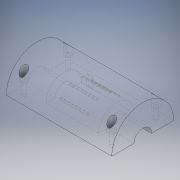
# Autodesk Inventor part: Slider Mount_C
Saved by Autodesk Inventor 2018 (Build 220112000, 112)
## iProperties
Created: 2018-01-08
Part Number: Slider Mount_C
Material: Generic
Document SubType Name: Modeling
Designer: njcfu
Density: 1 g/cm^3
Appearance: Default
Author: njcfu
Autodesk Inventor part; units mm, degrees
ref_plane "YZ Plane" through (0, 0, 0) normal (1, 0, 0) x (0, 1, 0)
ref_plane "XY Plane" through (0, 0, 0) normal (0, 0, 1) x (1, 0, 0)
sketch "Sketch1" plane through (0, 0, 0) normal (1, 0, 0) x (0, 1, 0)
  arc A0 (0, -25.4) -> (0, 25.4) centre (0, 0) ccw
  arc A1 (0, -44.45) -> (0, 44.45) centre (0, 0) ccw
  line L0 (0, 44.45) -> (0, 25.4)
  line L1 (0, -25.4) -> (0, -44.45)
  dimension "d24" = 25.4
  dimension "d27" = 44.45
  dimension "d29" = 0
  dimension "d32" = 19.05
  constraints: 4 end point, 4 point on circle, 2 centre point, 2 coincident, 1 collinear, 1 vertical
  measures "d24" distance of A0.centre L0.end
  measures "d27" radius of A1
  measures "d29" distance from line of point (0, 0) L1
  measures "d32" distance of L0.start L0.end
extrude "Extrusion1" add sketch "Sketch1" along normal mid plane 49.9999
ref_plane "Work Plane2" through (0, 25.4, 0) normal (0, 1, 0) x (-1, 0, 0)
sketch "Sketch3" plane through (0, 25.4, 0) normal (0, 1, 0) x (-1, 0, 0)
  point P0 (0, 0)
sketch "Sketch4" plane through (0, 25.4, 0) normal (0, 1, 0) x (-1, 0, 0)
  line L0 (3.3655, 0.9525) -> (-3.3655, 0.9525)
  line L1 (-3.3655, 0.9525) -> (-3.3655, -0.9525)
  line L2 (-3.3655, -0.9525) -> (3.3655, -0.9525)
  line L3 (3.3655, -0.9525) -> (3.3655, 0.9525)
  line L4 (3.3655, 0.9525) -> (-3.3655, -0.9525) construction
  line L5 (-3.3655, 0.9525) -> (3.3655, -0.9525) construction
  point P0 (0, 0)
  dimension "d30" = 6.731
  dimension "d31" = 1.905
  constraints: 12 end point, 2 midpoint, 2 parallel, 1 horizontal, 1 perpendicular
  measures "d30" distance of L1.end L2.end
  measures "d31" distance of L2.end L0.start
extrude "Extrusion3" cut sketch "Sketch4" along normal blind 14.986 and the other way blind 1.27
sketch "Sketch5" plane through (-25, 0, 0) normal (-1, 0, 0) x (0, 0, 1)
  arc A0 (44.45, 0) -> (-44.45, 0) centre (0, 0) ccw
  arc A1 (25.4, 0) -> (-25.4, 0) centre (0, 0) ccw
  arc A2 (44.45, 0) -> (-44.45, 0) centre (0, 0) ccw projected
  line L0 (-44.45, 0) -> (-25.4, 0) projected
  line L1 (-44.45, 0) -> (-25.4, 0)
  line L2 (25.4, 0) -> (44.45, 0)
  dimension "d40" = 19.05
  constraints: 4 end point, 4 point on circle, 2 centre point, 2 coincident, 2 collinear
  measures "d40" distance of L2.start L2.end
extrude "Extrusion4" add sketch "Sketch5" along normal blind 12.7
sketch "Sketch6" plane through (25, 0, 0) normal (1, 0, 0) x (0, 0, -1)
  arc A0 (44.45, 0) -> (-44.45, 0) centre (0, 0) ccw
  arc A1 (25.4, 0) -> (-25.4, 0) centre (0, 0) ccw
  line L0 (-44.45, 0) -> (-25.4, 0)
  line L1 (25.4, 0) -> (44.45, 0)
  dimension "d43" = 44.45
  dimension "d44" = 25.4
  dimension "d45" = 19.05
  dimension "d46" = 19.05
  constraints: 4 end point, 4 point on circle, 2 centre point, 2 coincident, 2 horizontal
  measures "d43" radius of A0
  measures "d44" radius of A1
  measures "d45" distance of L0.start L0.end
  measures "d46" distance of L1.start L1.end
extrude "Extrusion5" add sketch "Sketch6" along normal blind 12.7
sketch "Sketch7" plane through (-37.7, 0, 0) normal (-1, 0, 0) x (0, 0, 1)
  arc A0 (44.45, 0) -> (-44.45, 0) centre (0, 0) ccw
  arc A1 (12.7, 0) -> (-12.7, 0) centre (0, 0) ccw
  line L0 (-44.45, 0) -> (-12.7, 0)
  line L1 (12.7, 0) -> (44.45, 0)
  dimension "d49" = 44.45
  dimension "d50" = 12.7
  dimension "d51" = 31.75
  constraints: 4 end point, 4 point on circle, 2 centre point, 2 coincident, 2 point on line, 1 horizontal
  measures "d49" radius of A0
  measures "d50" radius of A1
  measures "d51" distance of L0.start L0.end
extrude "Extrusion6" add sketch "Sketch7" along normal blind 38.1
sketch "Sketch8" plane through (0, 0, 0) normal (1, 0, 0) x (0, 1, 0)
  line L0 (0, 0) -> (12.7, 21.997)
  line L1 (12.7, 21.997) -> (13.7999, 21.362)
  line L2 (13.7999, 21.362) -> (14.4349, 22.4619)
  line L3 (14.4349, 22.4619) -> (12.2351, 23.7319)
  line L4 (12.2351, 23.7319) -> (11.6001, 22.632)
  line L5 (11.6001, 22.632) -> (12.7, 21.997)
  line L6 (11.6001, 22.632) -> (11.2826, 22.0821)
  line L7 (11.2826, 22.0821) -> (13.4824, 20.8121)
  line L8 (13.4824, 20.8121) -> (13.7999, 21.362)
  line L9 (0, -12.7) -> (0, -25.4) projected
  dimension "d55" = 2.54
  dimension "d56" = 1.27
  dimension "d57" = 0.635
  dimension "d58" = 1.27
  dimension "d59" = 210
  dimension "d60" = 25.4
  constraints: 18 end point, 7 perpendicular, 1 collinear
  measures "d55" distance of L6.end L7.end
  measures "d56" distance between parallel lines of L0 L6
  measures "d57" distance between parallel lines of L7 L5
  measures "d58" distance between parallel lines of L5 L3
  measures "d60" distance of L0.start L0.end
extrude "Extrusion7" cut sketch "Sketch8" along normal mid plane 39.9999
pattern_circular "Circular Pattern2" count 4 over 120 about axis through (-10, 0, 0) along (-1, 0, 0) of "Extrusion7"
fillet "Fillet5" radius 0.254 8 edges at (0, 12.2351, -23.7319) (0, 14.4349, -22.4619) (0, 24.6272, -10.3151) (0, 25.496, -7.9283) (0, 25.496, 7.9283) (0, 24.6272, 10.3151) (0, 14.4349, 22.4619) (0, 12.2351, 23.7319)
sketch "Sketch9" plane through (37.7, 0, 0) normal (1, 0, 0) x (0, 0, -1)
  arc A0 (44.45, 0) -> (-44.45, 0) centre (0, 0) ccw
  arc A1 (12.7, 0) -> (-12.7, 0) centre (0, 0) ccw
  line L0 (-44.45, 0) -> (-12.7, 0)
  line L1 (12.7, 0) -> (44.45, 0)
  dimension "d67" = 44.45
  dimension "d68" = 12.7
  dimension "d69" = 31.75
  dimension "d70" = 12.7
  dimension "d71" = 44.45
  constraints: 4 end point, 4 point on circle, 2 centre point, 2 coincident, 2 point on line, 1 horizontal
  measures "d67" radius of A0
  measures "d68" radius of A1
  measures "d69" distance of L0.start L0.end
  measures "d70" distance of L0.end point (0, 0)
  measures "d71" distance of L1.end point (0, 0)
extrude "Extrusion8" add sketch "Sketch9" along normal blind 38.1
sketch "Sketch10" plane through (-37.7, 0, 12.7) normal (0, -1, 0) x (1, 0, 0)
  circle A0 centre (100.7999, 19.05) radius 2.413
  circle A1 centre (100.7999, -44.45) radius 2.413
  circle A2 centre (-25.4, -44.45) radius 2.413
  circle A3 centre (-25.4, 19.05) radius 2.413
  line L0 (113.4999, 31.75) -> (113.4999, 0) projected
  line L1 (-38.1, 31.75) -> (113.4999, 31.75) projected
  line L2 (-38.1, -57.15) -> (113.4999, -57.15) projected
  line L3 (113.4999, -25.4) -> (113.4999, -57.15) projected
  line L4 (-38.1, 0) -> (-38.1, 31.75) projected
  line L5 (-38.1, -57.15) -> (-38.1, -25.4) projected
  point P0 (37.6999, -12.7)
  dimension "d74" = 4.826
  dimension "d75" = 12.7
  dimension "d76" = 12.7
  dimension "d77" = 12.7
  dimension "d78" = 12.7
  dimension "d79" = 4.826
  dimension "d80" = 12.7
  dimension "d81" = 12.7
  dimension "d82" = 12.7
  dimension "d83" = 12.7
  dimension "d84" = 4.826
  dimension "d85" = 4.826
  constraints: 4 centre point
  measures "d74" diameter of A0
  measures "d75" distance from line of L0 A0.centre
  measures "d76" distance from line of L1 A0.centre
  measures "d77" distance from line of L2 A1.centre
  measures "d78" distance from line of L3 A1.centre
  measures "d79" diameter of A1
  measures "d80" distance from line of L1 A3.centre
  measures "d81" distance from line of L4 A3.centre
  measures "d82" distance from line of L5 A2.centre
  measures "d83" distance from line of L2 A2.centre
  measures "d84" diameter of A2
  measures "d85" diameter of A3
extrude "Extrusion9" cut sketch "Sketch10" against normal blind 38.1
ref_plane "Work Plane3" through (-37.7, 28.4375, 12.7) normal (0, -1, 0) x (1, 0, 0)
sketch "Sketch11" plane through (-37.7, 28.4375, 12.7) normal (0, -1, 0) x (1, 0, 0)
  circle A0 centre (-25.4, 19.05) radius 5.08
  circle A1 centre (100.7999, 19.05) radius 5.0759
  circle A2 centre (100.7999, -44.45) radius 5.08
  circle A3 centre (-25.4, -44.45) radius 5.08
  circle A4 centre (-25.4, 19.05) radius 2.413 projected
  circle A5 centre (-25.4, -44.45) radius 2.413 projected
  circle A6 centre (100.7999, -44.45) radius 2.413 projected
  circle A7 centre (100.7999, 19.05) radius 2.413 projected
  point P0 (37.6999, -12.7)
  dimension "d89" = 10.16
  dimension "d90" = 10.1518
  dimension "d91" = 10.16
  dimension "d92" = 10.16
  constraints: 4 centre point, 4 concentric
  measures "d89" diameter of A2
  measures "d90" diameter of A1
  measures "d91" diameter of A0
  measures "d92" diameter of A3
extrude "Extrusion10" cut sketch "Sketch11" along normal blind 10.16 and the other way blind 12.7
body "Solid1"
